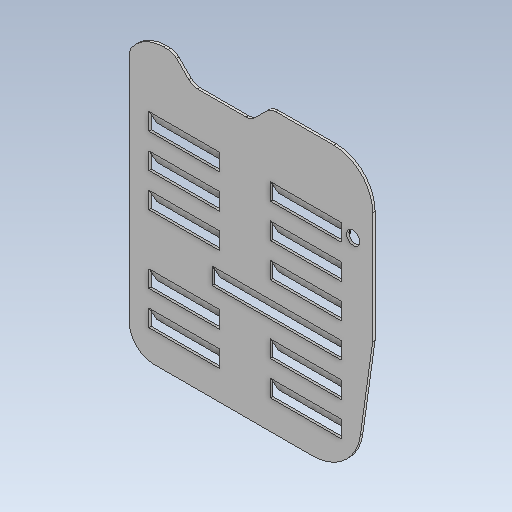
# Autodesk Inventor part: 65. Грязеуловитель
Saved by Autodesk Inventor 2021 (Build 250183000, 183)
## iProperties
Created: 2021-03-10
Part Number: 65. Грязеуловитель
Material: Типовые
Document SubType Name: Modeling
Designer: Данил
Density: 1 g/cm^3
Appearance: По умолчанию
Author: Данил
Autodesk Inventor part; units mm, degrees
ref_plane "YZ Plane" through (0, 0, 0) normal (1, 0, 0) x (0, 1, 0)
ref_plane "XZ Plane" through (0, 0, 0) normal (0, 1, 0) x (-1, 0, 0)
ref_plane "XY Plane" through (0, 0, 0) normal (0, 0, 1) x (1, 0, 0)
sketch "Эскиз1" plane through (0, 0, 0) normal (0, 0, 1) x (1, 0, 0)
  line L0 (-57.5, 0) -> (57.5, 0) construction
  line L1 (0, 57.5) -> (0, -57.5) construction
  line L2 (-37.5, -57.5) -> (32.6656, -57.5)
  line L3 (-57.5, -37.5) -> (-57.5, 7.6404)
  arc A0 (-57.5, -37.5) -> (-37.5, -57.5) centre (-37.5, -37.5) ccw
  arc A1 (-53.6765, 12.5) -> (-57.5, 7.6404) centre (-52.5, 7.6404) ccw
  arc A2 (-53.6765, 12.5) -> (-44.5, 24.1631) centre (-56.5, 24.1631) ccw
  line L4 (-44.5, 24.1631) -> (-44.5, 41.5)
  line L5 (-28.5, 57.5) -> (-26.6421, 57.5)
  arc A3 (-28.5, 57.5) -> (-44.5, 41.5) centre (-28.5, 41.5) ccw
  line L6 (-23.1066, 56.0355) -> (-18.0355, 50.9645)
  line L7 (-14.5, 49.5) -> (5.5, 49.5)
  line L8 (9.0355, 50.9645) -> (14.1066, 56.0355)
  line L9 (17.6421, 57.5) -> (41.5, 57.5)
  line L10 (57.5, 41.5) -> (57.5, -4.5)
  arc A4 (-23.1066, 56.0355) -> (-26.6421, 57.5) centre (-26.6421, 52.5) ccw
  arc A5 (-18.0355, 50.9645) -> (-14.5, 49.5) centre (-14.5, 54.5) ccw
  arc A6 (5.5, 49.5) -> (9.0355, 50.9645) centre (5.5, 54.5) ccw
  arc A7 (17.6421, 57.5) -> (14.1066, 56.0355) centre (17.6421, 52.5) ccw
  arc A8 (57.5, 41.5) -> (41.5, 57.5) centre (41.5, 41.5) ccw
  circle A9 centre (49.5, 28.5) radius 2.75
  line L11 (57.5, -4.5) -> (52.471, -40.2835)
  arc A10 (32.6656, -57.5) -> (52.471, -40.2835) centre (32.6656, -37.5) ccw
  line L12 (15.5, 31.5) -> (44.5, 31.5)
  line L13 (44.5, 31.5) -> (44.5, 24.5)
  line L14 (44.5, 24.5) -> (15.5, 24.5)
  line L15 (15.5, 24.5) -> (15.5, 31.5)
  line L16 (15.5, 17.5) -> (44.5, 17.5)
  line L17 (44.5, 17.5) -> (44.5, 10.5)
  line L18 (44.5, 10.5) -> (15.5, 10.5)
  line L19 (15.5, 10.5) -> (15.5, 17.5)
  line L20 (15.5, 3.5) -> (44.5, 3.5)
  line L21 (44.5, 3.5) -> (44.5, -3.5)
  line L22 (44.5, -3.5) -> (15.5, -3.5)
  line L23 (15.5, -3.5) -> (15.5, 3.5)
  line L24 (-5.5, 31.5) -> (-5.5, 24.5)
  line L25 (-5.5, 17.5) -> (-5.5, 10.5)
  line L26 (-34.5, 31.5) -> (-5.5, 31.5)
  line L27 (-34.5, 24.5) -> (-34.5, 31.5)
  line L28 (-5.5, 24.5) -> (-34.5, 24.5)
  line L29 (-34.5, 17.5) -> (-5.5, 17.5)
  line L30 (-34.5, 10.5) -> (-34.5, 17.5)
  line L31 (-5.5, 10.5) -> (-34.5, 10.5)
  line L32 (-34.5, 3.5) -> (-5.5, 3.5)
  line L33 (-5.5, -3.5) -> (-34.5, -3.5)
  line L34 (-34.5, -3.5) -> (-34.5, 3.5)
  line L35 (-5.5, 3.5) -> (-5.5, -3.5)
  line L36 (-34.5, -31.5) -> (-34.5, -24.5)
  line L37 (-34.5, -45.5) -> (-34.5, -38.5)
  line L38 (-5.5, -31.5) -> (-34.5, -31.5)
  line L39 (-34.5, -24.5) -> (-5.5, -24.5)
  line L40 (-34.5, -38.5) -> (-5.5, -38.5)
  line L41 (-5.5, -45.5) -> (-34.5, -45.5)
  line L42 (-5.5, -38.5) -> (-5.5, -45.5)
  line L43 (-5.5, -24.5) -> (-5.5, -31.5)
  line L44 (44.5, -24.5) -> (44.5, -31.5)
  line L45 (44.5, -38.5) -> (44.5, -45.5)
  line L46 (15.5, -45.5) -> (15.5, -38.5)
  line L47 (44.5, -45.5) -> (15.5, -45.5)
  line L48 (15.5, -38.5) -> (44.5, -38.5)
  line L49 (44.5, -31.5) -> (15.5, -31.5)
  line L50 (15.5, -31.5) -> (15.5, -24.5)
  line L51 (15.5, -24.5) -> (44.5, -24.5)
  line L52 (-8.5, -10.5) -> (44.5, -10.5)
  line L53 (44.5, -10.5) -> (44.5, -17.5)
  line L54 (44.5, -17.5) -> (-8.5, -17.5)
  line L55 (-8.5, -17.5) -> (-8.5, -10.5)
  point P0 (0, 0)
  point P1 (0, 0)
  point P2 (-57.5, -57.5)
  point P3 (-44.5, 57.5)
  point P4 (0, -42)
  dimension "d0" = 115
  dimension "d1" = 20
  dimension "d6" = 13
  dimension "d7" = 5
  dimension "d8" = 12
  dimension "d9" = 45
  dimension "d10" = 16
  dimension "d11" = 5
  dimension "d12" = 45
  dimension "d13" = 45
  dimension "d14" = 20
  dimension "d15" = 8
  dimension "d16" = 16
  dimension "d17" = 52
  dimension "d18" = 5.5
  dimension "d19" = 8
  dimension "d20" = 29
  dimension "d21" = 8
  dimension "d22" = 53
  dimension "d23" = 20
  dimension "d24" = 29
  dimension "d25" = 7
  dimension "d26" = 26
  dimension "d27" = 73
  dimension "d30" = 14
  dimension "d37" = 50
  dimension "d44" = 42
  dimension "d49" = 53
  dimension "d50" = 7
  dimension "d51" = 14
  constraints: 112 end point, 20 point on circle, 19 tangent, 11 centre point, 6 horizontal, 5 parallel, 5 perpendicular, 5 vertical, 4 point on line, 3 equal radius, 3 horizontal alignment, 3 vertical alignment, 2 midpoint, 1 coincident, 73 other
  measures "d0" distance of L0.start L0.end
  measures "d1" radius of A0
  measures "d6" distance between parallel lines of L3 L4
  measures "d7" radius of A1
  measures "d8" radius of A2
  measures "d9" vertical distance of point (-44.5, 57.5) A1.start
  measures "d10" radius of A3
  measures "d11" radius of A4
  measures "d12" angle of L7 L8
  measures "d13" angle of L7 L6
  measures "d14" distance of L7.start L7.end
  measures "d15" distance between parallel lines of L9 L7
  measures "d16" radius of A8
  measures "d17" distance from line of L10 L7.end
  measures "d18" diameter of A9
  measures "d19" distance from line of L10 A9.centre
  measures "d20" distance from line of L9 A9.centre
  measures "d21" angle of L10 L11
  measures "d22" distance from line of L2 L10.end
  measures "d23" radius of A10
  measures "d24" distance of L12.start L12.end
  measures "d25" distance of L12.end L13.end
  measures "d26" distance from line of L9 L12.end
  measures "d27" distance from line of L3 L14.end
  measures "d30" distance of L12.start L16.start
  measures "d37" distance of L12.end L24.start
  measures "d44" distance of L29.start L36.end
  measures "d49" distance of L52.start L52.end
  measures "d50" distance of L52.end L53.end
  measures "d51" distance from line of L52 L32.end
extrude "Выдавливание1" add sketch "Эскиз1" along normal mid plane 1
sketch "Эскиз2" plane through (44.5, 24.5, 0.5) normal (-1, 0, 0) x (0, 0, 1)
  line L0 (-1, 7) -> (0, 7) projected
  line L1 (0, 7) -> (0, 0) projected
  line L2 (0, 7) -> (-3.3141, 1.2598)
  line L3 (-3.7239, 1.15) -> (-3.9543, 1.283)
  line L4 (-1, 0) -> (-1, 7) projected
  line L5 (-4.0641, 1.6928) -> (-1, 7)
  line L6 (0, -29) -> (0, 17) projected
  arc A0 (-3.7239, 1.15) -> (-3.3141, 1.2598) centre (-3.5739, 1.4098) ccw
  arc A1 (-4.0641, 1.6928) -> (-3.9543, 1.283) centre (-3.8043, 1.5428) ccw
  point P0 (-0.5, -24.5)
  point P1 (-3.4641, 1)
  dimension "d54" = 30
  dimension "d55" = 6
  dimension "d56" = 0.3
  constraints: 6 end point, 4 point on circle, 4 tangent, 2 centre point, 2 point on line, 1 equal radius, 1 parallel, 1 perpendicular
  measures "d54" angle of L6 L2
  measures "d55" vertical distance of L0.end point (-3.464, 1)
  measures "d56" radius of A0
extrude "Выдавливание2" add sketch "Эскиз2" along normal up to surface (29 mm away)
pattern_linear "Прямоуг.массив1" count 2 spacing 50 along (-1, 0, 0) of "Выдавливание2"
pattern_linear "Прямоуг.массив2" count 3 spacing 14 along (0, -1, 0) of "Выдавливание2", "Прямоуг.массив1"
pattern_linear "Прямоуг.массив3" count 2 spacing 56 along (0, -1, 0) of "Выдавливание2", "Прямоуг.массив1"
pattern_linear "Прямоуг.массив4" count 2 spacing 70 along (0, -1, 0) of "Выдавливание2", "Прямоуг.массив1"
sketch "Эскиз3" plane through (44.5, -17.5, 0.5) normal (-1, 0, 0) x (0, 0, 1)
  line L0 (-1, 7) -> (0, 7) projected
  line L1 (0, 7) -> (0, 0) projected
  line L2 (0, 7) -> (-3.3141, 1.2598)
  line L3 (-3.7239, 1.15) -> (-3.9543, 1.283)
  line L4 (-4.0641, 1.6928) -> (-1, 7)
  arc A0 (-3.7239, 1.15) -> (-3.3141, 1.2598) centre (-3.5739, 1.4098) ccw
  arc A1 (-4.0641, 1.6928) -> (-3.9543, 1.283) centre (-3.8043, 1.5428) ccw
  point P0 (-0.5, 17.5)
  point P1 (-3.4641, 1)
  dimension "d71" = 30
  dimension "d72" = 6
  dimension "d73" = 0.3
  constraints: 6 end point, 4 point on circle, 4 tangent, 2 centre point, 2 point on line, 1 equal radius, 1 parallel, 1 perpendicular
  measures "d71" angle of L1 L2
  measures "d72" vertical distance of L0.end point (-3.464, 1)
  measures "d73" radius of A0
extrude "Выдавливание3" add sketch "Эскиз3" along normal up to surface (53 mm away)
sketch "Эскиз4" plane through (0, 0, 0.5) normal (0, 0, 1) x (1, 0, 0)
  line L0 (-44.5, 41.5) -> (-44.5, 24.1631) projected
  line L1 (-37.5, -57.5) -> (32.6656, -57.5) projected
  line L2 (-44.5, 24.1631) -> (-44.5, -57.5)
  arc A0 (-57.5, -37.5) -> (-37.5, -57.5) centre (-37.5, -37.5) ccw projected
  line L3 (-44.5, -57.5) -> (-37.5, -57.5)
  arc A1 (-53.6765, 12.5) -> (-44.5, 24.1631) centre (-56.5, 24.1631) ccw projected
  arc A2 (-53.6765, 12.5) -> (-57.5, 7.6404) centre (-52.5, 7.6404) ccw projected
  line L4 (-57.5, 7.6404) -> (-57.5, -37.5) projected
  point P0 (0, 0)
  point P1 (-44.5, -56.235)
  constraints: 4 end point, 1 collinear, 1 tangent, 1 vertical
extrude "Выдавливание4" cut sketch "Эскиз4" against normal through all contours L2 A0 L4 A2 A1
fillet "Сопряжение1" radius 10 1 edges at (-44.5, -56.235, 0)
sketch "Эскиз5" plane through (0, 0, 0.5) normal (0, 0, 1) x (1, 0, 0)
  line L0 (-42.5, -53.5) -> (-42.5, 49.246)
  line L1 (-44.5, 41.5) -> (-44.5, -47.5) projected
  arc A0 (-44.5, -47.5) -> (-34.5, -57.5) centre (-34.5, -47.5) ccw projected
  arc A1 (-28.5, 57.5) -> (-44.5, 41.5) centre (-28.5, 41.5) ccw projected
  point P0 (0, 0)
  dimension "d79" = 2
  constraints: 2 end point, 2 point on circle, 1 vertical
  measures "d79" distance between parallel lines of L1 L0
extrude "Выдавливание5" cut sketch "Эскиз5" against normal through all
fillet "Сопряжение2" radius 10 1 edges at (-42.5, -53.5, 0)
fillet "Сопряжение3" radius 5 1 edges at (-42.5, 49.246, 0)
